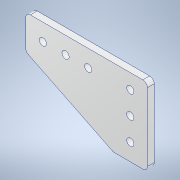
# Autodesk Inventor part: オムニ_koteigu
Saved by Autodesk Inventor 2021 (Build 250183000, 183)
## iProperties
Created: 2022-02-03
Part Number: オムニ_koteigu
Material: アルミニウム 6061
Document SubType Name: Modeling
Designer: hirohumi
Density: 2.7 g/cm^3
Appearance: アルミニウム - フラット
Author: hirohumi
Autodesk Inventor part; units mm, degrees
ref_plane "YZ Plane" through (0, 0, 0) normal (1, 0, 0) x (0, 1, 0)
ref_plane "XZ Plane" through (0, 0, 0) normal (0, 1, 0) x (-1, 0, 0)
ref_plane "作業平面1" through (0, 0, 0) normal (0, 0, 1) x (1, 0, 0)
sketch "スケッチ1" plane through (0, 0, 0) normal (0, 0, 1) x (1, 0, 0)
  circle A0 centre (7.5, 170) radius 1.6 projected
  circle A1 centre (7.5, 180) radius 1.6 projected
  circle A2 centre (7.5, 190) radius 1.6 projected
  circle A3 centre (-11.0383, 189) radius 1.6 projected
  circle A4 centre (-21.0383, 189) radius 1.6 projected
  circle A5 centre (-31.0383, 189) radius 1.6 projected
  line L0 (15, 162.5) -> (0, 162.5)
  line L1 (0, 162.5) -> (-38.5383, 181.5)
  line L2 (-38.5383, 181.5) -> (-38.5383, 196.5)
  line L3 (-38.5383, 196.5) -> (15, 196.5)
  line L4 (15, 196.5) -> (15, 162.5)
  point P0 (0, 0)
  dimension "d0" = 7.5
  dimension "d1" = 7.5
  dimension "d2" = 7.5
  dimension "d3" = 7.5
  dimension "d4" = 7.5
  dimension "d5" = 7.5
  constraints: 10 end point, 2 perpendicular, 1 horizontal, 1 vertical
  measures "d0" distance from line of A5.centre L2
  measures "d1" distance from line of A0.centre L0
  measures "d2" distance from line of L3 A3.centre
  measures "d3" distance from line of A2.centre L4
  measures "d4" horizontal distance of A0.centre L0.end
  measures "d5" horizontal distance of A5.centre L1.end
extrude "押し出し1" add sketch "スケッチ1" along normal blind 3
fillet "フィレット1" radius 2 5 edges at (15, 162.5, 1.5) (15, 196.5, 1.5) (-38.5383, 196.5, 1.5) (-38.5383, 181.5, 1.5) (0, 162.5, 1.5)
